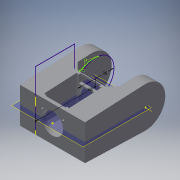
# Autodesk Inventor part: knuckle1
Saved by Autodesk Inventor 2018 (Build 220112000, 112)
## iProperties
Created: 2018-02-01
Part Number: knuckle1
Material: Generic
Document SubType Name: Modeling
Designer: Clevo
Density: 1 g/cm^3
Appearance: Default
Author: Clevo
Autodesk Inventor part; units mm, degrees
ref_plane "YZ Plane" through (0, 0, 0) normal (1, 0, 0) x (0, 1, 0)
ref_plane "XZ Plane" through (0, 0, 0) normal (0, 1, 0) x (-1, 0, 0)
ref_plane "XY Plane" through (0, 0, 0) normal (0, 0, 1) x (1, 0, 0)
sketch "Sketch1" plane through (0, 0, 0) normal (0, 1, 0) x (-1, 0, 0)
  line L0 (12.25, 22.5) -> (-12.25, 22.5)
  line L1 (-12.25, 22.5) -> (-12.25, -22.5)
  line L2 (-12.25, -22.5) -> (12.25, -22.5)
  line L3 (12.25, -22.5) -> (12.25, 22.5)
  point P0 (0, 0)
  point P1 (12.25, 0)
  point P2 (0, 22.5)
  dimension "d0" = 24.5
  dimension "d1" = 45
  constraints: 8 end point, 2 midpoint, 2 parallel, 1 horizontal, 1 horizontal alignment, 1 perpendicular, 1 vertical alignment
  measures "d0" distance of L2.end L1.end
  measures "d1" distance of L1.end L0.end
extrude "Extrusion1" add sketch "Sketch1" along normal blind 1.95
sketch "Sketch2" plane through (0, 1.95, 0) normal (0, 1, 0) x (1, 0, 0)
  line L0 (-10, 1.25) -> (10, 1.25)
  line L1 (10, 1.25) -> (10, -17.25)
  line L2 (10, -17.25) -> (-10, -17.25)
  line L3 (-10, -17.25) -> (-10, 1.25)
  line L4 (-12.25, -22.5) -> (12.25, -22.5) projected
  line L5 (12.25, -22.5) -> (12.25, 22.5) projected
  line L6 (12.25, 22.5) -> (-12.25, 22.5) projected
  line L7 (-12.25, 22.5) -> (-12.25, -22.5) projected
  line L8 (-7, -17.25) -> (7, -17.25)
  line L9 (7, -17.25) -> (7, -22.5)
  line L10 (7, -22.5) -> (-7, -22.5)
  line L11 (-7, -22.5) -> (-7, -17.25)
  line L12 (-12.25, -22.5) -> (12.25, -22.5) projected
  point P0 (0, 0)
  dimension "d4" = 2.25
  dimension "d5" = 20
  dimension "d6" = 2.25
  dimension "d7" = 5.25
  dimension "d8" = 5.25
  dimension "d9" = 14
  dimension "d10" = 5.25
  dimension "d11" = 18.5
  constraints: 16 end point, 4 parallel, 2 horizontal, 2 perpendicular, 1 collinear, 1 point on line
  measures "d4" distance between parallel lines of L7 L3
  measures "d5" distance of L0.start L0.end
  measures "d6" distance between parallel lines of L5 L1
  measures "d7" distance of L8.end L9.end
  measures "d8" distance between parallel lines of L7 L11
  measures "d9" distance between parallel lines of L9 L11
  measures "d10" distance between parallel lines of L5 L9
  measures "d11" distance of L0.end L1.end
extrude "Extrusion2" cut sketch "Sketch2" against normal up to surface (1.95 mm away) contours L0 L1 L2 L3 | L2 L9 L4 L11
sketch "Sketch3" plane through (0, 1.95, 0) normal (0, 1, 0) x (1, 0, 0)
  line L0 (-7, -22.5) -> (-7, -17.25) projected
  line L1 (-7, -17.25) -> (-10, -17.25) projected
  line L2 (-10, -17.25) -> (-10, 1.25) projected
  line L3 (-10, 1.25) -> (10, 1.25) projected
  line L4 (10, 1.25) -> (10, -17.25) projected
  line L5 (10, -17.25) -> (7, -17.25) projected
  line L6 (7, -17.25) -> (7, -22.5) projected
  line L7 (7, -22.5) -> (12.25, -22.5) projected
  line L8 (12.25, -22.5) -> (12.25, 22.5) projected
  line L9 (12.25, 22.5) -> (-12.25, 22.5) projected
  line L10 (-12.25, 22.5) -> (-12.25, -22.5) projected
  line L11 (-12.25, -22.5) -> (-7, -22.5) projected
  point P0 (0, 0)
  point P1 (-10.25, -20.305)
  point P2 (10.25, -20.305)
  dimension "d14" = 20.5
  dimension "d15" = 2
  dimension "d16" = 2.195
  dimension "d17" = 2
  constraints: 1 horizontal alignment
  measures "d14" distance of point (10.25, -20.305) point (-10.25, -20.305)
  measures "d15" distance from line of L8 point (10.25, -20.305)
  measures "d16" distance from line of L11 point (-10.25, -20.305)
  measures "d17" distance from line of L10 point (-10.25, -20.305)
hole "Hole1" at (-10.25, 1.95, 20.305) at (10.25, 1.95, 20.305) direction (0, -1, 0) diameter 2.4 end through all clearance for "Flat Head Machine Screw" size "M2" standard "Ansi Metric M Profile"
sketch "Sketch4" plane through (0, 1.95, 0) normal (0, 1, 0) x (1, 0, 0)
  circle A0 centre (-10.25, -20.305) radius 1.2 projected
  circle A1 centre (10.25, -20.305) radius 1.2 projected
  line L0 (-7, -22.5) -> (-7, -17.25) projected
  line L1 (-7, -17.25) -> (-10, -17.25) projected
  line L2 (-10, -17.25) -> (-10, 1.25) projected
  line L3 (-10, 1.25) -> (10, 1.25) projected
  line L4 (10, 1.25) -> (10, -17.25) projected
  line L5 (10, -17.25) -> (7, -17.25) projected
  line L6 (7, -17.25) -> (7, -22.5) projected
  line L7 (7, -22.5) -> (12.25, -22.5) projected
  line L8 (12.25, -22.5) -> (12.25, 22.5) projected
  line L9 (12.25, 22.5) -> (-12.25, 22.5) projected
  line L10 (-12.25, 22.5) -> (-12.25, -22.5) projected
  line L11 (-12.25, -22.5) -> (-7, -22.5) projected
  point P0 (0, 0)
  point P1 (-10.25, 4.15)
  point P2 (10.25, 4.15)
  dimension "d25" = 20.5
  dimension "d26" = 26.65
  dimension "d27" = 2
  dimension "d28" = 2
  constraints: 1 horizontal alignment
  measures "d25" distance of point (10.25, 4.15) point (-10.25, 4.15)
  measures "d26" distance from line of L11 point (-10.25, 4.15)
  measures "d27" distance from line of L10 point (-10.25, 4.15)
  measures "d28" distance from line of L8 point (10.25, 4.15)
hole "Hole2" at (-10.25, 1.95, -4.15) at (10.25, 1.95, -4.15) direction (0, -1, 0) diameter 2.4 end through all clearance for "Flat Head Machine Screw" size "M2" standard "Ansi Metric M Profile"
fillet "Fillet1" radius 0.5 2 edges at (7, 0.975, 17.25) (-7, 0.975, 17.25)
sketch "Sketch5" plane through (0, 1.95, 0) normal (0, 1, 0) x (1, 0, 0)
  circle A0 centre (-10.25, 4.15) radius 1.2 projected
  circle A1 centre (10.25, 4.15) radius 1.2 projected
  circle A2 centre (-10.25, -20.305) radius 1.2 projected
  circle A3 centre (10.25, -20.305) radius 1.2 projected
  arc A4 (-7, -17.75) -> (-7.5, -17.25) centre (-7.5, -17.75) ccw projected
  line L0 (-7.5, -17.25) -> (-10, -17.25) projected
  line L1 (-10, -17.25) -> (-10, 1.25) projected
  line L2 (-10, 1.25) -> (10, 1.25) projected
  line L3 (10, 1.25) -> (10, -17.25) projected
  line L4 (10, -17.25) -> (7.5, -17.25) projected
  arc A5 (7.5, -17.25) -> (7, -17.75) centre (7.5, -17.75) ccw projected
  line L5 (7, -17.75) -> (7, -22.5) projected
  line L6 (7, -22.5) -> (12.25, -22.5) projected
  line L7 (12.25, -22.5) -> (12.25, 22.5) projected
  line L8 (12.25, 22.5) -> (-12.25, 22.5) projected
  line L9 (-12.25, 22.5) -> (-12.25, -22.5) projected
  line L10 (-12.25, -22.5) -> (-7, -22.5) projected
  line L11 (-7, -22.5) -> (-7, -17.75) projected
  line L12 (-12.25, 22.5) -> (-12.25, -22.5) projected
  line L13 (12.25, -22.5) -> (12.25, 22.5) projected
  line L14 (-12.25, -22.5) -> (12.25, -22.5)
  line L15 (12.25, -22.5) -> (12.25, -4.5)
  line L16 (12.25, -4.5) -> (10, -4.5)
  line L17 (-12.25, -4.5) -> (-12.25, -22.5)
  line L18 (-10, -4.5) -> (-12.25, -4.5)
  line L19 (10, -4.5) -> (-10, -4.5)
  point P0 (0, 0)
  dimension "d37" = 18
  constraints: 12 end point, 4 parallel, 3 point on line, 1 horizontal, 1 perpendicular
  measures "d37" distance between parallel lines of L14 L16
extrude "Extrusion3" add sketch "Sketch5" along normal blind 1 contours L11 L10 L9 L18 L1 L0 A4 | A4 L0 L1 L19 L3 L4 A5 L5 L14 L11 | L5 A5 L4 L3 L16 L7 L6 | L18 L9 L8 L7 L16 L3 L2 L1
sketch "Sketch6" plane through (12.25, 0, 22.5) normal (1, 0, 0) x (0, 0, -1)
  line L0 (0, 0) -> (45, 0) projected
  line L1 (45, 0) -> (45, 2.95) projected
  line L2 (0, 2.95) -> (45, 2.95) projected
  line L3 (0, 0) -> (0, 2.95) projected
  line L4 (45, 0) -> (45, 2.95) projected
  line L5 (45, 2.95) -> (0, 2.95)
  line L6 (0, 2.95) -> (0, -32)
  line L7 (0, -32) -> (45, -32)
  line L8 (45, -32) -> (45, 2.95)
  line L9 (0, 0) -> (0, 2.95) projected
  line L10 (0, 0) -> (45, 0) projected
  line L11 (45, 0) -> (0, 0)
  line L12 (0, 0) -> (0, -32)
  line L13 (0, -32) -> (45, -32)
  line L14 (45, -32) -> (45, 0)
  point P0 (22.5, 0)
  dimension "d72" = 32
  constraints: 16 end point, 4 parallel, 2 horizontal, 2 perpendicular, 1 collinear
  measures "d72" distance between parallel lines of L0 L7
extrude "Extrusion4" add sketch "Sketch6" along normal blind 5
sketch "Sketch7" plane through (12.25, -32, -22.5) normal (0, -1, 0) x (1, 0, 0)
  line L0 (0, 45) -> (0, 0) projected
  line L1 (0, 0) -> (5, 0) projected
  line L2 (5, 45) -> (5, 0) projected
  line L3 (0, 45) -> (5, 45) projected
  line L4 (0, 0) -> (-24.5, 0) projected
  line L5 (0, 0) -> (-24.5, 0)
  line L6 (-24.5, 0) -> (-24.5, 45)
  line L7 (-24.5, 45) -> (0, 45)
  line L8 (0, 45) -> (0, 0)
  point P0 (-12.25, 22.5)
  dimension "d43" = 24.5
  constraints: 8 end point, 2 parallel, 1 collinear, 1 horizontal, 1 perpendicular
  measures "d43" distance of L0.end L5.end
extrude "Extrusion5" add sketch "Sketch7" along normal blind 1.15
sketch "Sketch8" plane through (12.25, -33.15, -22.5) normal (0, -1, 0) x (1, 0, 0)
  line L0 (-24.5, 0) -> (5, 0) projected
  line L1 (5, 0) -> (5, 45) projected
  line L2 (5, 45) -> (-24.5, 45) projected
  line L3 (-24.5, 45) -> (-24.5, 0) projected
  circle A0 centre (-12.25, 10) radius 10.5
  line L4 (-19.25, 45) -> (-5.25, 45) projected
  line L5 (-5, 45) -> (-19.5, 45)
  line L6 (-19.5, 45) -> (-19.5, 36)
  line L7 (-19.5, 36) -> (-5, 36)
  line L8 (-5, 36) -> (-5, 45)
  line L9 (-2.25, 21.25) -> (-22.25, 21.25)
  line L10 (-22.25, 21.25) -> (-22.25, 36)
  line L11 (-22.25, 36) -> (-2.25, 36)
  line L12 (-2.25, 36) -> (-2.25, 21.25)
  line L13 (-5, 21.25) -> (-19.5, 21.25)
  line L14 (-19.5, 21.25) -> (-19.5, 17.25)
  line L15 (-19.5, 17.25) -> (-5, 17.25)
  line L16 (-5, 17.25) -> (-5, 21.25)
  line L17 (-24.5, 0) -> (5, 0) projected
  line L18 (-24.5, 45) -> (0, 45)
  line L19 (0, 45) -> (0, 0)
  line L20 (0, 0) -> (-24.5, 0)
  line L21 (-24.5, 0) -> (-24.5, 45)
  point P0 (-12.25, 22.5)
  dimension "d46" = 10
  dimension "d47" = 21
  dimension "d48" = 14.5
  dimension "d49" = 20
  dimension "d50" = 14.5
  dimension "d51" = 24.5
  dimension "d52" = 5
  dimension "d53" = 5
  dimension "d54" = 2.25
  dimension "d55" = 2.25
  dimension "d56" = 5
  dimension "d57" = 5
  dimension "d58" = 9
  dimension "d59" = 14.75
  dimension "d60" = 4
  constraints: 32 end point, 8 parallel, 4 horizontal, 4 perpendicular, 4 point on line, 1 centre point, 1 vertical alignment
  measures "d46" distance from line of L0 A0.centre
  measures "d47" diameter of A0
  measures "d48" distance between parallel lines of L6 L8
  measures "d49" distance of L10.end L11.end
  measures "d50" distance of L14.end L15.end
  measures "d51" distance between parallel lines of L3 L19
  measures "d52" distance between parallel lines of L19 L16
  measures "d53" distance between parallel lines of L3 L14
  measures "d54" distance between parallel lines of L19 L12
  measures "d55" distance between parallel lines of L3 L10
  measures "d56" distance between parallel lines of L3 L6
  measures "d57" distance between parallel lines of L19 L8
  measures "d58" distance of L5.end L6.end
  measures "d59" distance of L9.end L10.end
  measures "d60" distance of L13.end L14.end
extrude "Extrusion6" cut sketch "Sketch8" against normal up to surface (1.15 mm away) contours A0 L0 | L0 A0 L14 L15 L16 | L8 L7 L6 L2 | L14 L9 L16 A0 | A0 L16 L15 L14 | L11 L12 L9 L10 L7
sketch "Sketch9" plane through (12.25, -33.15, -22.5) normal (0, -1, 0) x (1, 0, 0)
  line L0 (-5, 45) -> (-5, 36) projected
  line L1 (-5, 36) -> (-2.25, 36) projected
  line L2 (-2.25, 36) -> (-2.25, 21.25) projected
  line L3 (-2.25, 21.25) -> (-5, 21.25) projected
  line L4 (-5, 21.25) -> (-5, 17.5952) projected
  arc A0 (-9.0484, 0) -> (-5, 17.5952) centre (-12.25, 10) ccw projected
  line L5 (-9.0484, 0) -> (5, 0) projected
  line L6 (5, 0) -> (5, 45) projected
  line L7 (5, 45) -> (-5, 45) projected
  line L8 (-19.5, 36) -> (-19.5, 45) projected
  line L9 (-19.5, 45) -> (-24.5, 45) projected
  line L10 (-24.5, 45) -> (-24.5, 0) projected
  line L11 (-24.5, 0) -> (-15.4516, 0) projected
  arc A1 (-19.5, 17.5952) -> (-15.4516, 0) centre (-12.25, 10) ccw projected
  line L12 (-19.5, 17.5952) -> (-19.5, 21.25) projected
  line L13 (-19.5, 21.25) -> (-22.25, 21.25) projected
  line L14 (-22.25, 21.25) -> (-22.25, 36) projected
  line L15 (-22.25, 36) -> (-19.5, 36) projected
  circle A2 centre (-22.5, 18.35) radius 1.2 projected
  circle A3 centre (-2, 18.35) radius 1.2 projected
  circle A4 centre (-2, 42.805) radius 1.2 projected
  circle A5 centre (-22.5, 42.805) radius 1.2 projected
  line L16 (-2, 18.35) -> (-22.5, 18.35)
  line L17 (-22.5, 18.35) -> (-22.5, 39.05)
  line L18 (-22.5, 39.05) -> (-2, 39.05)
  line L19 (-2, 39.05) -> (-2, 18.35)
  point P0 (-12.25, 22.5)
  dimension "d63" = 20.7
  constraints: 8 end point, 2 parallel, 1 horizontal, 1 perpendicular, 1 point on line
  measures "d63" distance of L16.end L17.end
hole "Hole3" at (-10.25, -33.15, -4.15) at (10.25, -33.15, -4.15) at (10.25, -33.15, 16.55) at (-10.25, -33.15, 16.55) direction (0, 1, 0) diameter 2.4 depth 8 tip angle 118 clearance for "Flat Head Machine Screw" size "M2" standard "Ansi Metric M Profile"
sketch "Sketch10" plane through (12.25, -33.15, -22.5) normal (0, -1, 0) x (1, 0, 0)
  circle A0 centre (-2, 39.05) radius 1.2 projected
  circle A1 centre (-2, 18.35) radius 1.2 projected
  line L0 (-5, 45) -> (-5, 36) projected
  line L1 (-5, 36) -> (-2.25, 36) projected
  line L2 (-2.25, 36) -> (-2.25, 21.25) projected
  line L3 (-2.25, 21.25) -> (-5, 21.25) projected
  line L4 (-5, 21.25) -> (-5, 17.5952) projected
  arc A2 (-9.0484, 0) -> (-5, 17.5952) centre (-12.25, 10) ccw projected
  line L5 (-9.0484, 0) -> (5, 0) projected
  line L6 (5, 0) -> (5, 45) projected
  line L7 (5, 45) -> (-5, 45) projected
  circle A3 centre (-22.5, 18.35) radius 1.2 projected
  circle A4 centre (-22.5, 39.05) radius 1.2 projected
  line L8 (-19.5, 36) -> (-19.5, 45) projected
  line L9 (-19.5, 45) -> (-24.5, 45) projected
  line L10 (-24.5, 45) -> (-24.5, 0) projected
  line L11 (-24.5, 0) -> (-15.4516, 0) projected
  arc A5 (-19.5, 17.5952) -> (-15.4516, 0) centre (-12.25, 10) ccw projected
  line L12 (-19.5, 17.5952) -> (-19.5, 21.25) projected
  line L13 (-19.5, 21.25) -> (-22.25, 21.25) projected
  line L14 (-22.25, 21.25) -> (-22.25, 36) projected
  line L15 (-22.25, 36) -> (-19.5, 36) projected
  line L16 (5, 0) -> (5, 45) projected
  line L17 (-24.5, 0) -> (-24.5, 45) projected
  line L18 (5, 0) -> (-24.5, 0)
  line L19 (-24.5, 0) -> (-24.5, 45)
  line L20 (-24.5, 45) -> (5, 45)
  line L21 (5, 45) -> (5, 0)
  arc A6 (-19.5, 17.5952) -> (-15.4516, 0) centre (-12.25, 10) ccw projected
  circle A7 centre (-12.25, 10) radius 10.5
  point P0 (-12.25, 22.5)
  constraints: 8 end point, 2 parallel, 1 coincident, 1 horizontal, 1 perpendicular, 3 other
extrude "Extrusion7" add sketch "Sketch10" along normal blind 3
sketch "Sketch11" plane through (12.25, -36.15, -22.5) normal (0, -1, 0) x (1, 0, 0)
  line L0 (-9.0484, 0) -> (5, 0) projected
  line L1 (5, 0) -> (5, 45) projected
  line L2 (5, 45) -> (-24.5, 45) projected
  line L3 (-24.5, 45) -> (-24.5, 0) projected
  line L4 (-24.5, 0) -> (-15.4516, 0) projected
  arc A0 (-15.4516, 0) -> (-9.0484, 0) centre (-12.25, 10) ccw projected
  arc A1 (-19.5, 17.5952) -> (-15.4516, 0) centre (-12.25, 10) ccw projected
  circle A2 centre (-12.25, 10) radius 10.5
  point P0 (-12.25, 22.5)
  constraints: 1 coincident, 3 other
extrude "Extrusion8" cut sketch "Sketch11" against normal up to surface (3 mm away) contours A0 A1 A2
sketch "Sketch12" plane through (-12.25, 0, -22.5) normal (-1, 0, 0) x (0, 0, 1)
  line L0 (-6.0754, -39.5109) -> (50.3226, -39.5109)
  line L1 (50.3226, -39.5109) -> (50.3226, 16.733)
  line L2 (50.3226, 16.733) -> (-6.0754, 16.733)
  line L3 (-6.0754, 16.733) -> (-6.0754, -39.5109)
  point P0 (22.5, 0)
  constraints: 8 end point, 2 parallel, 1 horizontal, 1 perpendicular
extrude "Extrusion9" cut sketch "Sketch12" against normal blind 12.25
sketch "Sketch13" plane through (0, 0, 0) normal (0, -1, 0) x (1, 0, 0)
  arc A0 (3.2016, -22.5) -> (0, -2) centre (0, -12.5) ccw projected
  circle A1 centre (0, -12.5) radius 4
  point P0 (0, 0)
  dimension "d80" = 8
  constraints: 1 centre point, 1 coincident
  measures "d80" diameter of A1
extrude "Extrusion10" cut sketch "Sketch13" against normal blind 4.5
sketch "Sketch14" plane through (12.25, 0, 22.5) normal (-1, 0, 0) x (0, 0, 1)
  line L0 (0, 0) -> (-45, 0) projected
  line L1 (-45, -32) -> (-45, 0) projected
  line L2 (0, -32) -> (-45, -32) projected
  line L3 (0, 0) -> (0, -32) projected
  point P0 (-22.5, 0)
extrude "Extrusion11" cut sketch "Sketch14" against normal blind 0.2
sketch "Sketch16" plane through (17.25, -36.15, -22.5) normal (0, 0, -1) x (-1, 0, 0)
  line L0 (17.25, 39.1) -> (0, 39.1) projected
  line L1 (0, 39.1) -> (0, 0) projected
  line L2 (14.0484, 0) -> (0, 0) projected
  line L3 (14.0484, 4.15) -> (4.8, 4.15) projected
  line L4 (4.8, 4.15) -> (4.8, 36.15) projected
  line L5 (4.8, 36.15) -> (17.25, 36.15) projected
  line L6 (17.25, 39.1) -> (17.25, 38.1) projected
  line L7 (0, 0) -> (17.25, 0)
  line L8 (17.25, 0) -> (17.25, 39.1)
  line L9 (17.25, 39.1) -> (0, 39.1)
  line L10 (0, 39.1) -> (0, 0)
  line L11 (14.0484, 0) -> (14.0484, 4.15) projected
  line L12 (17.25, 36.15) -> (17.25, 39.1) projected
  constraints: 8 end point, 2 parallel, 1 horizontal, 1 perpendicular
extrude "Extrusion13" add sketch "Sketch16" along normal blind 8
sketch "Sketch17" plane through (7, 0, 22.5) normal (0, 0, 1) x (1, 0, 0)
  line L0 (0, 0) -> (5.45, 0) projected
  line L1 (5.45, 0) -> (5.45, -32) projected
  line L2 (5.45, -32) -> (0.25, -32) projected
  line L3 (0.25, -32) -> (0.25, -33.15) projected
  line L4 (0.25, -33.15) -> (-7, -33.15) projected
  line L5 (-7, -33.15) -> (-7, -36.15) projected
  line L6 (10.25, -36.15) -> (-7, -36.15) projected
  line L7 (10.25, 2.95) -> (10.25, -36.15) projected
  line L8 (-7, 2.95) -> (10.25, 2.95) projected
  line L9 (-7, 2.95) -> (-7, 1.95) projected
  line L10 (-7, 1.95) -> (0, 1.95) projected
  line L11 (0, 1.95) -> (0, 0) projected
  line L12 (-7, 2.95) -> (10.25, 2.95) projected
  line L13 (-7, -36.15) -> (-7, -33.15) projected
  line L14 (10.25, 2.95) -> (-7, 2.95)
  line L15 (-7, 2.95) -> (-7, -36.15)
  line L16 (-7, -36.15) -> (10.25, -36.15)
  line L17 (10.25, -36.15) -> (10.25, 2.95)
  point P0 (-7, 0)
  constraints: 8 end point, 2 parallel, 1 horizontal, 1 perpendicular
extrude "Extrusion14" add sketch "Sketch17" along normal blind 5
sketch "Sketch18" plane through (12.25, -36.15, -22.5) normal (0, -1, 0) x (1, 0, 0)
  line L0 (-12.25, 50) -> (-12.25, 20.5) projected
  arc A0 (-9.0484, 0) -> (-12.25, 20.5) centre (-12.25, 10) ccw projected
  line L1 (-9.0484, 0) -> (-12.25, 0) projected
  line L2 (-12.25, 0) -> (-12.25, -8) projected
  line L3 (5, -8) -> (-12.25, -8) projected
  line L4 (5, 50) -> (5, -8) projected
  line L5 (-12.25, 50) -> (5, 50) projected
  circle A1 centre (-2, 39.05) radius 1.2 projected
  circle A2 centre (-2, 18.35) radius 1.2 projected
  line L6 (-12.25, 21.25) -> (-12.25, 20.5) projected
  circle A3 centre (-12.25, 10) radius 10.5
  point P0 (-12.25, 22.5)
  constraints: 1 coincident, 1 vertical alignment, 2 other
extrude "Extrusion15" cut sketch "Sketch18" against normal up to surface (39.1 mm away) contours A0 L1 L2 A3 | L2 L1 A3
sketch "Sketch19" plane through (17.25, -36.15, -22.5) normal (0, 0, 1) x (1, 0, 0)
  line L0 (-14.0484, 36.15) -> (-14.0484, 4.15) projected
  line L1 (-14.0484, 4.15) -> (-4.8, 4.15) projected
  line L2 (-4.8, 4.15) -> (-4.8, 36.15) projected
  line L3 (-4.8, 36.15) -> (-14.0484, 36.15) projected
  line L4 (-4.8, 36.15) -> (-39.7398, 36.15)
  line L5 (-39.7398, 36.15) -> (-39.7398, 4.15)
  line L6 (-39.7398, 4.15) -> (-4.8, 4.15)
  line L7 (-4.8, 4.15) -> (-4.8, 36.15)
  point P0 (-17.25, 36.15)
  constraints: 8 end point, 2 parallel, 1 collinear, 1 horizontal, 1 perpendicular
extrude "Extrusion16" cut sketch "Sketch19" against normal blind 0.2
sketch "Sketch20" plane through (7, 0, 22.5) normal (0, 0, -1) x (-1, 0, 0)
  line L0 (-0.25, -33.15) -> (7, -33.15) projected
  line L1 (7, 1.95) -> (7, -33.15) projected
  line L2 (7, 1.95) -> (0, 1.95) projected
  line L3 (0, 1.95) -> (0, 0) projected
  line L4 (0, 0) -> (-5.45, 0) projected
  line L5 (-5.45, 0) -> (-5.45, -32) projected
  line L6 (-5.45, -32) -> (-0.25, -32) projected
  line L7 (-0.25, -32) -> (-0.25, -33.15) projected
  point P0 (7, 0)
extrude "Extrusion17" cut sketch "Sketch20" against normal blind 0.2
chamfer "Chamfer1" distance 2.5 angle 45 1 edges at (12.45, -16, -22.7)
fillet "Fillet7" radius 1.5 1 edges at (12.45, -16, 22.7)
fillet "Fillet8" radius 0.5 2 edges at (7.25, -32.575, -1.25) (7.25, -32.575, 13.5)
mirror "Mirror1" about plane through (0, -11.389, -0.3764) normal (-1, 0, 0)
sketch "Sketch26" plane through (-17.25, -36.15, -30.5) normal (-1, 0, 0) x (0, 0, 1)
  line L0 (28.5, 0) -> (7.5, 0)
  line L1 (18, 0) -> (18, 60)
  circle A0 centre (18, 60) radius 18
  line L2 (58, 39.1) -> (0, 39.1)
  line L3 (0, 39.1) -> (0, 0)
  line L4 (58, 0) -> (0, 0)
  line L5 (58, 0) -> (58, 39.1)
  line L6 (0, 39.1) -> (0, 0)
  line L7 (3.5997, 0) -> (3.5997, 13.0245) construction
  line L8 (-1.6612, 55.1559) -> (0.4915, 64.1777) construction
  spline S0 degree 3 poles (0, 33.0988) (-1.4544, 44.6685) (-1.6612, 55.1559) (0.4915, 64.1777) knots 1.476317 1.476317 1.476317 1.476317 2 2 2 2
  line L9 (32.4788, 39.1) -> (32.4788, 42.7786) construction
  line L10 (32.4788, 42.7786) -> (30.8189, 47.3637) construction
  line L11 (30.8189, 47.3637) -> (38.3833, 49.7592) construction
  line L12 (38.3833, 49.7592) -> (35.6557, 63.5038) construction
  spline S1 degree 4 poles (32.4788, 39.1) (32.4788, 42.7786) (30.8189, 47.3637) (38.3833, 49.7592) (35.6557, 63.5038) knots 1 1 1 1 1 2 2 2 2 2
  spline S2 degree 3 poles (3.5997, 0) (3.5997, 13.0245) (1.4311, 21.7144) (0, 33.0988) knots 0 0 0 0 1 1 1 1
  line L13 (3.5997, 13.0245) -> (1.4311, 21.7144) construction
  line L14 (1.4311, 21.7144) -> (0, 33.0988) construction
  line L15 (-1.4544, 44.6685) -> (-1.6612, 55.1559) construction
  line L16 (0, 33.0988) -> (-1.4544, 44.6685) construction
  line L17 (58, 0) -> (58, 39.1)
  line L18 (58, 0) -> (32.4788, 0)
  line L19 (32.4788, 0) -> (32.4788, 39.1)
  line L20 (32.4788, 39.1) -> (58, 39.1)
  line L21 (58, 39.1) -> (58, 0)
  line L22 (58, 0) -> (0, 0)
  line L23 (3.5997, 0) -> (24.308, 0)
  line L24 (24.308, 0) -> (24.308, 31)
  line L25 (24.308, 31) -> (3.5997, 31)
  line L26 (3.5997, 31) -> (3.5997, 0)
  point P0 (30.5, 36.15)
  dimension "d130" = 60
  dimension "d131" = 36
  constraints: 18 end point, 4 parallel, 3 point on circle, 3 point on line, 3 vertical, 2 horizontal, 2 perpendicular, 1 centre point, 1 coincident, 1 midpoint, 10 other
  measures "d130" distance of L1.start L1.end
  measures "d131" diameter of A0
sketch "Sketch31" plane through (-17.25, -36.15, -30.5) normal (-1, 0, 0) x (0, 0, 1)
  line L0 (58, 39.1) -> (0, 39.1) projected
  line L1 (0, 39.1) -> (0, 0) projected
  line L2 (58, 0) -> (0, 0) projected
  line L3 (58, 0) -> (58, 39.1) projected
  line L4 (28.5, 0) -> (7.5, 0) projected
  line L5 (8, 1.35) -> (28, 1.35) projected
  line L6 (18, 1.35) -> (18, 59.35)
  circle A0 centre (18, 59.35) radius 20
  line L7 (-1.9885, 58.6726) -> (-1.3252, 39.1)
  line L8 (58, 0) -> (0, 0) projected
  line L9 (-1.3252, 39.1) -> (0, 0)
  line L10 (35, 38.1) -> (35, 39.1) projected
  line L11 (37.9745, 58.341) -> (35.0274, 0)
  point P0 (30.5, 36.15)
  dimension "d146" = 40
  dimension "d147" = 58
  dimension "d148" = 0
  dimension "d149" = 2
  constraints: 8 end point, 3 point on line, 3 tangent, 2 point on circle, 1 centre point, 1 coincident, 1 midpoint, 1 vertical
  measures "d146" diameter of A0
  measures "d147" distance of L6.start L6.end
  measures "d148" distance of L1.end L9.end
  measures "d149" distance from line of L10.end L11
extrude "Extrusion24" add sketch "Sketch31" along normal blind 15 contours L11 L2 L1 L0 | L0 L6 A0 L11 | A0 | L0 L1 L9 L7 A0 L6
sketch "Sketch32" plane through (-32.25, -36.15, -30.5) normal (-1, 0, 0) x (0, 0, 1)
  line L0 (0, 0) -> (35.0274, 0) projected
  line L1 (35.0274, 0) -> (37.9745, 58.341) projected
  arc A0 (37.9745, 58.341) -> (-1.9885, 58.6726) centre (18, 59.35) ccw projected
  line L2 (-1.9885, 58.6726) -> (0, 0) projected
  point P0 (30.5, 36.15)
extrude "Extrusion25" cut sketch "Sketch32" against normal up to surface (49.5 mm away) keep common part
sketch "Sketch33" plane through (-17.25, -36.15, -30.5) normal (1, 0, 0) x (0, 0, -1)
  line L0 (0, 39.1) -> (0, 0) projected
  line L1 (1.9885, 58.6726) -> (0, 0) projected
  arc A0 (1.9885, 58.6726) -> (-37.9745, 58.341) centre (-18, 59.35) ccw projected
  line L2 (-37.0026, 39.1) -> (-37.9745, 58.341) projected
  line L3 (-37.0026, 39.1) -> (0, 39.1) projected
  point P0 (-30.5, 36.15)
extrude "Extrusion26" add sketch "Sketch33" along normal up to surface (34.5 mm away)
sketch "Sketch34" plane through (17.25, 0, 22.5) normal (1, 0, 0) x (0, 0, -1)
  line L0 (17.9726, -36.15) -> (15.0255, 22.191) projected
  line L1 (17.9726, -36.15) -> (53, -36.15) projected
  line L2 (54.9885, 22.5226) -> (53, -36.15) projected
  arc A0 (54.9885, 22.5226) -> (15.0255, 22.191) centre (35, 23.2) ccw projected
  point P0 (22.5, 0)
extrude "Extrusion27" add sketch "Sketch34" along normal blind 15
ref_plane "Work Plane2" through (-32.25, 23.2, -12.5) normal (0, 0, -1) x (1, 0, 0)
sketch "Sketch35" plane through (-32.25, 23.2, -12.5) normal (0, 0, -1) x (1, 0, 0)
  line L0 (11.5, 0) -> (53, 0)
  line L1 (53, 0) -> (53, 20.5)
  line L2 (53, 20.5) -> (11.5, 20.5)
  line L3 (11.5, 20.5) -> (11.5, 0)
  line L4 (77.4, 0) -> (-12.9, 0) projected
  line L5 (44.7, 55.2) -> (42.75, 55.2) projected
  line L6 (42.75, 55.2) -> (42.75, 59.35) projected
  line L7 (42.75, 59.35) -> (64.5, 59.35) projected
  line L8 (64.5, 59.35) -> (64.5, -20) projected
  line L9 (64.5, -20) -> (0, -20) projected
  line L10 (0, -20) -> (0, 59.35) projected
  line L11 (0, 59.35) -> (21.75, 59.35) projected
  line L12 (21.75, 59.35) -> (21.75, 55.2) projected
  line L13 (21.75, 55.2) -> (19.8, 55.2) projected
  line L14 (19.8, 55.2) -> (19.8, 23.2) projected
  line L15 (19.8, 23.2) -> (21.75, 23.2) projected
  line L16 (21.75, 23.2) -> (21.75, 20.25) projected
  line L17 (21.75, 20.25) -> (42.75, 20.25) projected
  line L18 (42.75, 20.25) -> (42.75, 23.2) projected
  line L19 (42.75, 23.2) -> (44.7, 23.2) projected
  line L20 (44.7, 23.2) -> (44.7, 55.2) projected
  line L21 (18.25, 20.5) -> (11.5, 13.5)
  line L22 (46.25, 20.5) -> (53, 13.5)
  point P0 (32.25, 23.2)
  point P1 (32.25, 20.5)
  point P2 (32.25, 20.25)
  dimension "d158" = 20.5
  dimension "d159" = 41.5
  dimension "d160" = 14
  dimension "d161" = 14
  dimension "d162" = 7
  constraints: 12 end point, 4 point on line, 2 midpoint, 2 parallel, 1 collinear, 1 horizontal, 1 horizontal alignment, 1 perpendicular, 1 vertical alignment
  measures "d158" distance of L2.end L0.start
  measures "d159" distance of L1.end L2.end
  measures "d160" distance of point (32.25, 20.5) L22.start
  measures "d161" distance of L21.start point (32.25, 20.5)
  measures "d162" distance from line of L2 L21.end
extrude "Extrusion28" cut sketch "Sketch35" along normal mid plane 100 contours L3 L21 L2 L16 L17 L18 L22 L1 L0 | L2 L18 L17 L16
sketch "Sketch37" plane through (-20.75, 23.2, -32.5) normal (0, -1, 0) x (1, 0, 0)
  line L0 (41.5, 0) -> (0, 0) projected
  line L1 (41.5, 40) -> (41.5, 0) projected
  line L2 (0, 40) -> (41.5, 40) projected
  line L3 (0, 0) -> (0, 40) projected
  point P0 (20.75, 32.5)
extrude "Extrusion29" cut sketch "Sketch37" against normal up to surface round surface about axis through (-17.25, 23.2, -12.5) along (-1, 0, 0) radius 20 far side no
chamfer "Chamfer2" distance 6 angle 45 3 edges at (0, 2.7, -31.8167) (-17.375, 6.2, -31.9353) (17.375, 6.2, -31.9353)
sketch "Sketch38" plane through (-32.25, 23.2, -12.5) normal (0, 0, -1) x (1, 0, 0)
  point P0 (32.25, 23.2)
equation "\"d4\" = d6"
equation "\"d8\" = d10"
equation "\"d15\" = d17"
equation "\"d27\" = d28"
equation "\"d52\" = d53"
equation "\"d54\" = d55"
equation "\"d56\" = d57"
body "Solid1"
